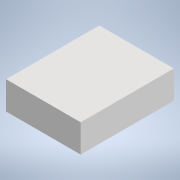
# Autodesk Inventor part: Metal Inside
Saved by Autodesk Inventor 2021 (Build 250183000, 183)
## iProperties
Created: 2020-11-29
Part Number: Metal Inside
Material: Generic
Document SubType Name: Modeling
Designer: deli
Density: 1 g/cm^3
Appearance: Default
Author: deli
Autodesk Inventor part; units mm, degrees
ref_plane "YZ Plane" through (0, 0, 0) normal (1, 0, 0) x (0, 1, 0)
ref_plane "XZ Plane" through (0, 0, 0) normal (0, 1, 0) x (-1, 0, 0)
ref_plane "XY Plane" through (0, 0, 0) normal (0, 0, 1) x (1, 0, 0)
sketch "Sketch1" plane through (0, 0, 0) normal (1, 0, 0) x (0, 1, 0)
  line L0 (22.5733, 37.2966) -> (14.6231, 37.2966)
  line L1 (14.6231, 37.2966) -> (14.6231, 5.5466)
  line L2 (14.6231, 5.5466) -> (22.5733, 5.5466)
  line L3 (22.5733, 5.5466) -> (22.5733, 37.2966)
  point P0 (0, 0)
  dimension "d0" = 7.9502
  dimension "d1" = 31.75
  constraints: 8 end point, 2 parallel, 1 horizontal, 1 perpendicular
  measures "d0" distance of L2.end L1.end
  measures "d1" distance of L1.end L0.end
extrude "Extrusion1" add sketch "Sketch1" along normal blind 25.4
sketch "Sketch2" plane through (0, 14.6231, 37.2966) normal (0, 0, 1) x (1, 0, 0)
  line L0 (0, 7.9502) -> (25.4, 7.9502) projected
  line L1 (25.4, 0) -> (15.24, 0)
  line L2 (15.24, 0) -> (15.24, 7.9502)
  line L3 (15.24, 7.9502) -> (25.4, 7.9502)
  line L4 (25.4, 7.9502) -> (25.4, 0)
  point P0 (0, -14.6231)
  dimension "d4" = 10.16
  constraints: 8 end point, 2 parallel, 1 horizontal, 1 perpendicular, 1 point on line
  measures "d4" distance of L2.end L3.end
extrude "Extrusion2" cut sketch "Sketch2" against normal blind 7.62
sketch "Sketch3" plane through (0, 14.6231, 29.6766) normal (0, 0, 1) x (1, 0, 0)
  line L0 (25.4, 7.9502) -> (25.4, 0) projected
  line L1 (15.24, 7.9502) -> (25.4, 7.9502) projected
  line L2 (15.24, 0) -> (15.24, 7.9502) projected
  line L3 (25.4, 0) -> (15.24, 0) projected
  circle A0 centre (20.32, 3.9502) radius 2
  point P0 (0, -14.6231)
  dimension "d7" = 4
  dimension "d10" = 4
  constraints: 1 centre point
  measures "d7" diameter of A0
  measures "d10" distance from line of L1 A0.centre
extrude "Extrusion3" cut sketch "Sketch3" against normal blind 2.54 contours A0
sketch "Sketch4" plane through (0, 22.5733, 37.2966) normal (0, 1, 0) x (1, 0, 0)
  circle A0 centre (10.16, 6.0198) radius 2
  line L0 (15.24, 0) -> (15.24, 7.62) projected
  line L1 (0, 0) -> (15.24, 0) projected
  point P0 (0, 37.2966)
  dimension "d11" = 4
  dimension "d12" = 5.08
  dimension "d15" = 6.0198
  constraints: 1 centre point
  measures "d11" diameter of A0
  measures "d12" distance from line of A0.centre L0
  measures "d15" distance from line of A0.centre L1
extrude "Extrusion4" cut sketch "Sketch4" against normal blind 25.4
sketch "Sketch5" plane through (0, 22.5733, 37.2966) normal (0, 1, 0) x (1, 0, 0)
  line L0 (0, 0) -> (15.24, 0) projected
  line L1 (0, 31.75) -> (25.4, 31.75) projected
  line L2 (14.605, 0) -> (5.715, 0)
  line L3 (5.715, 0) -> (5.715, 31.75)
  line L4 (5.715, 31.75) -> (14.605, 31.75)
  line L5 (14.605, 31.75) -> (14.605, 0)
  circle A0 centre (10.16, 6.0198) radius 2 projected
  point P0 (0, 37.2966)
  point P1 (5.715, 0)
  dimension "d16" = 8.89
  dimension "d17" = 4.445
  constraints: 8 end point, 2 parallel, 2 point on line, 1 horizontal, 1 perpendicular
  measures "d16" distance of L3.end L4.end
  measures "d17" distance from line of L3 A0.centre
extrude "Extrusion5" cut sketch "Sketch5" against normal blind 2.54
body "Solid1"
